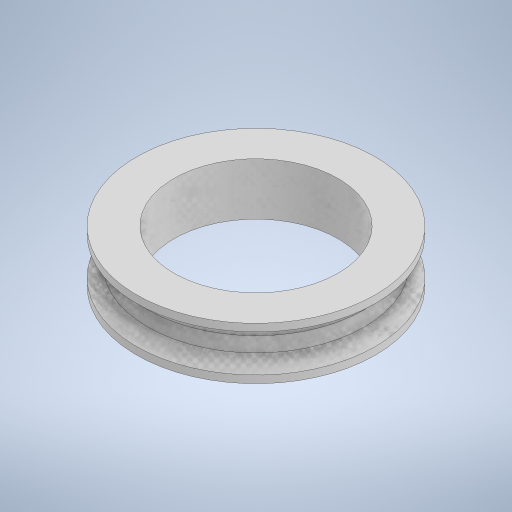
# Autodesk Inventor part: Polea
Saved by Autodesk Inventor 2024 (Build 280153000, 153)
## iProperties
Created: 2024-05-28
Part Number: Polea
Material: Genérico
Document SubType Name: Modeling
Designer: Elena Portas
Density: 1 g/cm^3
Appearance: Valor por defecto
Author: Elena Portas
## iProperties of the stored document Polea_3DPrint.ipt
Created: 2024-05-28
Part Number: Polea_3DPrint
Material: Genérico
Document SubType Name: Modeling
Designer: Elena Portas
Density: 1 g/cm^3
Appearance: Valor por defecto
Author: Elena Portas
Autodesk Inventor part; units mm, degrees
ref_plane "YZ Plane" through (0, 0, 0) normal (1, 0, 0) x (0, 1, 0)
ref_plane "XZ Plane" through (0, 0, 0) normal (0, 1, 0) x (-1, 0, 0)
ref_plane "XY Plane" through (0, 0, 0) normal (0, 0, 1) x (1, 0, 0)
sketch "Boceto1" plane through (0, 0, 0) normal (0, 0, 1) x (1, 0, 0)
  line L0 (11, 3.5) -> (11, -3.5)
  line L1 (11, 3.5) -> (16, 3.5)
  line L2 (16, 3.5) -> (16, 2.5)
  line L3 (16, 2.5) -> (14.5, 1)
  line L4 (14.5, 1) -> (14.5, 0)
  line L5 (11, -3.5) -> (16, -3.5)
  line L6 (16, -3.5) -> (16, -2.5)
  line L7 (16, -2.5) -> (14.5, -1)
  line L8 (14.5, -1) -> (14.5, 0)
  line L9 (0, 4.9) -> (0, -4.9) projected
  line L10 (0, -4.9) -> (0, 4.9) projected
  point P0 (0, 0)
  dimension "d2" = 5
  dimension "d3" = 1
  dimension "d4" = 135
  dimension "d5" = 1.5
  dimension "d6" = 7
  dimension "d7" = 11
  constraints: 18 end point, 2 vertical, 1 horizontal
  measures "d2" distance of L0.start L1.end
  measures "d3" distance of L1.end L2.end
  measures "d4" angle of L2 L3
  measures "d5" horizontal distance of L2.end L3.end
  measures "d6" distance between parallel lines of L5 L1
  measures "d7" distance between parallel lines of L0 L9
revolve "Revolución1" add sketch "Boceto1" angle 360 about axis through (0, -10, 0) along (0, 1, 0)
